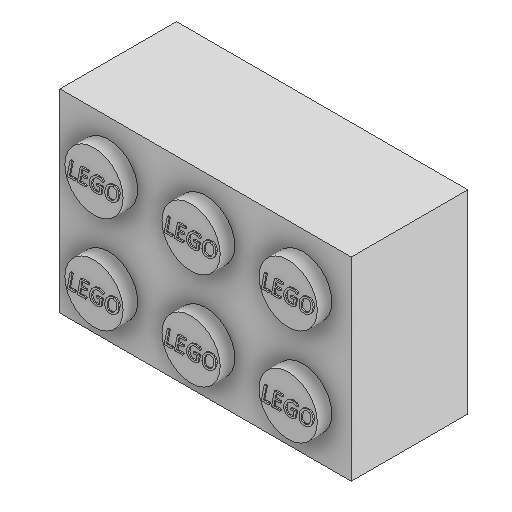
# Autodesk Inventor part: LEGO 2x4 Brick
Saved by Autodesk Inventor 2026.2 (Build 302298000, 298)
## iProperties
Created: 2026-01-06
Part Number: LEGO 2x4 Brick
Material: Generic
Document SubType Name: Modeling
Designer: andyeske
Density: 1 g/cm^3
Appearance: Default
Author: andyeske
Autodesk Inventor part; units mm, degrees
ref_plane "YZ Plane" through (0, 0, 0) normal (1, 0, 0) x (0, 1, 0)
ref_plane "XZ Plane" through (0, 0, 0) normal (0, 1, 0) x (-1, 0, 0)
ref_plane "XY Plane" through (0, 0, 0) normal (0, 0, 1) x (1, 0, 0)
sketch "Sketch1" plane through (0, 0, 0) normal (0, 0, 1) x (1, 0, 0)
  line L0 (-12, -8) -> (12, -8)
  line L1 (12, -8) -> (12, 8)
  line L2 (12, 8) -> (-12, 8)
  line L3 (-12, 8) -> (-12, -8)
  line L4 (-12, -8) -> (12, 8) construction
  line L5 (12, -8) -> (-12, 8) construction
  point P0 (0, 0)
  dimension "d0" = 24
  dimension "d1" = 16
  constraints: 12 end point, 2 midpoint, 2 parallel, 1 horizontal, 1 perpendicular
  measures "d0" distance of L1.end L2.end
  measures "d1" distance of L0.end L1.end
extrude "Extrusion1" add sketch "Sketch1" along normal blind 9.6
shell "Shell1" thickness 1.2 removed faces 1 at (4, -2.6667, 0)
sketch "Sketch2" plane through (0, 0, 9.6) normal (0, 0, 1) x (1, 0, 0)
  line L0 (-12, 4) -> (-8, 4) construction
  line L1 (-8, 4) -> (-8, 8) construction
  line L2 (-12, 8) -> (-12, -8) projected
  line L3 (12, 8) -> (-12, 8) projected
  circle A0 centre (-8, 4) radius 2.4
  point P0 (0, 0)
  dimension "d5" = 4
  dimension "d6" = 4
  dimension "d7" = 4.8
  constraints: 4 end point, 2 point on line, 1 centre point, 1 coincident, 1 horizontal, 1 perpendicular
  measures "d5" distance of L0.end L1.end
  measures "d6" distance of L0.start L0.end
  measures "d7" diameter of A0
extrude "Extrusion2" add sketch "Sketch2" along normal blind 1.2
sketch "Sketch3" plane through (-8, 4, 10.8) normal (0, 0, 1) x (1, 0, 0)
  circle A0 centre (0, 0) radius 2.4 projected
  line L0 (-2.3103, -0.65) -> (2.3103, -0.65) construction
  line L1 (0, 0) -> (0, -0.65) construction
  spline S0 degree 2 poles (-1.4435, -0.5379) (-1.4435, -0.5427) (-1.4459, -0.5641) (-1.4519, -0.5892) (-1.4578, -0.6154) (-1.4697, -0.6369) (-1.4852, -0.65) (-1.4948, -0.65) knots 0 0 0 1 2 3 4 5 6 6 6
  line L2 (-1.4948, -0.65) -> (-2.0553, -0.65)
  spline S1 degree 2 poles (-2.0553, -0.65) (-2.0672, -0.65) (-2.0875, -0.6428) (-2.103, -0.6262) (-2.1089, -0.5999) (-2.1041, -0.582) knots 0 0 0 1 2 3 4 4 4
  line L3 (-2.1041, -0.582) -> (-1.8704, 0.5902)
  spline S2 degree 2 poles (-1.8704, 0.5902) (-1.8692, 0.5962) (-1.8573, 0.6081) (-1.8358, 0.6152) (-1.8024, 0.62) (-1.7798, 0.62) knots 0 0 0 1 2 3 4 4 4
  spline S3 degree 2 poles (-1.7798, 0.62) (-1.7559, 0.62) (-1.7237, 0.6152) (-1.7059, 0.6081) (-1.6999, 0.5962) (-1.7023, 0.5902) knots 0 0 0 1 2 3 4 4 4
  line L4 (-1.7023, 0.5902) -> (-1.9205, -0.5045)
  line L5 (-1.9205, -0.5045) -> (-1.4674, -0.5045)
  spline S4 degree 2 poles (-1.4674, -0.5045) (-1.4542, -0.5045) (-1.4435, -0.5224) (-1.4435, -0.5379) knots 0 0 0 1 2 2 2
  spline S5 degree 2 poles (-0.3405, 0.5818) (-0.3405, 0.5771) (-0.3416, 0.5568) (-0.3464, 0.5329) (-0.3536, 0.5079) (-0.3643, 0.4876) (-0.381, 0.4745) (-0.3917, 0.4745) knots 0 0 0 1 2 3 4 5 6 6 6
  line L6 (-0.3917, 0.4745) -> (-0.8842, 0.4745)
  line L7 (-0.8842, 0.4745) -> (-0.9641, 0.0774)
  line L8 (-0.9641, 0.0774) -> (-0.5396, 0.0774)
  spline S6 degree 2 poles (-0.5396, 0.0774) (-0.5277, 0.0774) (-0.5158, 0.0619) (-0.5158, 0.0464) knots 0 0 0 1 2 2 2
  spline S7 degree 2 poles (-0.5158, 0.0464) (-0.5158, 0.0416) (-0.5181, 0.0202) (-0.5229, -0.0037) (-0.5301, -0.0275) (-0.5408, -0.0454) (-0.5563, -0.0585) (-0.567, -0.0585) knots 0 0 0 1 2 3 4 5 6 6 6
  line L9 (-0.567, -0.0585) -> (-0.9916, -0.0585)
  line L10 (-0.9916, -0.0585) -> (-1.0822, -0.5105)
  line L11 (-1.0822, -0.5105) -> (-0.5801, -0.5105)
  spline S8 degree 2 poles (-0.5801, -0.5105) (-0.5706, -0.5105) (-0.5575, -0.526) (-0.5575, -0.5427) knots 0 0 0 1 2 2 2
  spline S9 degree 2 poles (-0.5575, -0.5427) (-0.5575, -0.5486) (-0.5599, -0.5701) (-0.5646, -0.594) (-0.5706, -0.6178) (-0.5825, -0.6381) (-0.5992, -0.65) (-0.6088, -0.65) knots 0 0 0 1 2 3 4 5 6 6 6
  line L12 (-0.6088, -0.65) -> (-1.2169, -0.65)
  spline S10 degree 2 poles (-1.2169, -0.65) (-1.2277, -0.65) (-1.2479, -0.6428) (-1.2622, -0.6262) (-1.2682, -0.5999) (-1.2634, -0.582) knots 0 0 0 1 2 3 4 4 4
  line L13 (-1.2634, -0.582) -> (-1.0381, 0.5461)
  spline S11 degree 2 poles (-1.0381, 0.5461) (-1.0309, 0.5842) (-0.9844, 0.614) (-0.9617, 0.614) knots 0 0 0 1 2 2 2
  line L14 (-0.9617, 0.614) -> (-0.3631, 0.614)
  spline S12 degree 2 poles (-0.3631, 0.614) (-0.3405, 0.614) (-0.3405, 0.5818) knots 0 0 0 1 1 1
  spline S13 degree 2 poles (0.8723, 0.4769) (0.8723, 0.4697) (0.8699, 0.4495) (0.864, 0.4268) (0.8568, 0.403) (0.8473, 0.3839) (0.8353, 0.3732) (0.8282, 0.3732) knots 0 0 0 1 2 3 4 5 6 6 6
  spline S14 degree 2 poles (0.8282, 0.3732) (0.8139, 0.3732) (0.7638, 0.4089) (0.6803, 0.4531) (0.5611, 0.4888) (0.4788, 0.4888) knots 0 0 0 1 2 3 4 4 4
  spline S15 degree 2 poles (0.4788, 0.4888) (0.3917, 0.4888) (0.2403, 0.4375) (0.1127, 0.3457) (0.0137, 0.2217) (-0.0566, 0.0762) (-0.0924, -0.0836) (-0.0924, -0.1658) knots 0 0 0 1 2 3 4 5 6 6 6
  spline S16 degree 2 poles (-0.0924, -0.1658) (-0.0924, -0.2517) (-0.0423, -0.3841) (0.0519, -0.4735) (0.1842, -0.52) (0.2665, -0.52) knots 0 0 0 1 2 3 4 4 4
  spline S17 degree 2 poles (0.2665, -0.52) (0.3273, -0.52) (0.4585, -0.4914) (0.5158, -0.4628) knots 0 0 0 1 2 2 2
  line L15 (0.5158, -0.4628) -> (0.5885, -0.0967)
  line L16 (0.5885, -0.0967) -> (0.2963, -0.0967)
  spline S18 degree 2 poles (0.2963, -0.0967) (0.2856, -0.0967) (0.2725, -0.08) (0.2725, -0.0645) knots 0 0 0 1 2 2 2
  spline S19 degree 2 poles (0.2725, -0.0645) (0.2725, -0.0573) (0.2749, -0.0347) (0.2808, -0.0108) (0.2892, 0.0118) (0.3011, 0.0309) (0.3154, 0.0416) (0.3238, 0.0416) knots 0 0 0 1 2 3 4 5 6 6 6
  line L17 (0.3238, 0.0416) -> (0.7256, 0.0416)
  spline S20 degree 2 poles (0.7256, 0.0416) (0.7531, 0.0416) (0.7769, 0.0047) (0.7709, -0.0263) knots 0 0 0 1 2 2 2
  line L18 (0.7709, -0.0263) -> (0.6732, -0.5141)
  spline S21 degree 2 poles (0.6732, -0.5141) (0.6696, -0.5319) (0.6565, -0.5546) (0.6493, -0.5629) knots 0 0 0 1 2 2 2
  spline S22 degree 2 poles (0.6493, -0.5629) (0.6398, -0.5725) (0.5682, -0.6059) (0.4597, -0.6417) (0.3238, -0.6679) (0.2498, -0.6679) knots 0 0 0 1 2 3 4 4 4
  spline S23 degree 2 poles (0.2498, -0.6679) (0.1222, -0.6679) (-0.071, -0.6023) (-0.2021, -0.4771) (-0.2701, -0.2994) (-0.2701, -0.1873) knots 0 0 0 1 2 3 4 4 4
  spline S24 degree 2 poles (-0.2701, -0.1873) (-0.2701, -0.0824) (-0.2224, 0.1203) (-0.1318, 0.3016) (-0.0006, 0.4554) (0.1711, 0.5675) (0.3762, 0.6319) (0.4955, 0.6319) knots 0 0 0 1 2 3 4 5 6 6 6
  spline S25 degree 2 poles (0.4955, 0.6319) (0.5635, 0.6319) (0.6827, 0.6081) (0.7769, 0.5735) (0.8413, 0.5329) (0.864, 0.5115) (0.8723, 0.4912) (0.8723, 0.4769) knots 0 0 0 1 2 3 4 5 6 6 6
  spline S26 degree 2 poles (2.153, 0.1907) (2.153, 0.1156) (2.1256, -0.0705) (2.0612, -0.2624) (1.9551, -0.4437) (1.7989, -0.5832) (1.5842, -0.6691) (1.4447, -0.6691) knots 0 0 0 1 2 3 4 5 6 6 6
  spline S27 degree 2 poles (1.4447, -0.6691) (1.3338, -0.6691) (1.1657, -0.613) (1.0536, -0.5033) (0.9963, -0.3411) (0.9963, -0.2338) knots 0 0 0 1 2 3 4 4 4
  spline S28 degree 2 poles (0.9963, -0.2338) (0.9963, -0.1503) (1.0261, 0.044) (1.0929, 0.236) (1.2014, 0.4137) (1.3588, 0.552) (1.5699, 0.6331) (1.707, 0.6331) knots 0 0 0 1 2 3 4 5 6 6 6
  spline S29 degree 2 poles (1.707, 0.6331) (1.8179, 0.6331) (1.9837, 0.5759) (2.097, 0.4626) (2.153, 0.298) (2.153, 0.1907) knots 0 0 0 1 2 3 4 4 4
  spline S30 degree 2 poles (1.973, 0.1788) (1.973, 0.2479) (1.942, 0.3624) (1.874, 0.4435) (1.7607, 0.49) (1.6808, 0.49) knots 0 0 0 1 2 3 4 4 4
  spline S31 degree 2 poles (1.6808, 0.49) (1.5795, 0.49) (1.4256, 0.4149) (1.3135, 0.2933) (1.2396, 0.1394) (1.1967, -0.0168) (1.1776, -0.1635) (1.1776, -0.2171) knots 0 0 0 1 2 3 4 5 6 6 6
  spline S32 degree 2 poles (1.1776, -0.2171) (1.1776, -0.2863) (1.2074, -0.3996) (1.2778, -0.4795) (1.391, -0.5236) (1.4721, -0.5236) knots 0 0 0 1 2 3 4 4 4
  spline S33 degree 2 poles (1.4721, -0.5236) (1.5723, -0.5236) (1.7237, -0.4497) (1.8358, -0.3304) (1.9098, -0.179) (1.9539, -0.0239) (1.973, 0.1227) (1.973, 0.1788) knots 0 0 0 1 2 3 4 5 6 6 6
  point P0 (8, -4)
  dimension "d10" = 0.65
  constraints: 4 end point, 2 horizontal, 2 point on circle, 1 midpoint
  measures "d10" distance of L1.start L1.end
extrude "Extrusion3" add sketch "Sketch3" along normal blind 0.1 contours S0 L2 S1 L3 S2 S3 L4 L5 S4 | S5 L6 L7 L8 S6 S7 L9 L10 L11 S8 S9 L12 S10 L13 S11 L14 S12 | S13 S14 S15 S16 S17 L15 L16 S18 S19 L17 S20 L18 S21 S22 S23 S24 S25 | S26 S27 S28 S29
sketch "Sketch4" plane through (10.8, -6.8, 8.4) normal (0, 0, -1) x (-1, 0, 0)
  circle A0 centre (18.8, 10.8) radius 2.4 construction
  circle A1 centre (18.8, 10.8) radius 1.2
  point P0 (10.8, 6.8)
  dimension "d13" = 1.2
  constraints: 1 centre point, 1 coincident
  measures "d13" radial gap between concentric circles of A0 A1
extrude "Extrusion4" cut sketch "Sketch4" against normal blind 1.2
pattern_linear "Rectangular Pattern1" count 3 spacing 8 along (1, 0, 0) count 2 spacing 8 along (0, -1, 0) of "Extrusion3", "Extrusion2", "Extrusion4"
sketch "Sketch5" plane through (10.8, -6.8, 8.4) normal (0, 0, -1) x (-1, 0, 0)
  line L0 (21.6, 13.6) -> (21.6, 0) projected
  line L1 (21.6, 6.8) -> (14.8, 6.8) construction
  line L2 (14.8, 6.8) -> (14.8, 0) construction
  line L3 (21.6, 0) -> (0, 0) projected
  circle A0 centre (14.8, 6.8) radius 3.2
  circle A1 centre (14.8, 6.8) radius 2.6
  point P0 (10.8, 6.8)
  dimension "d22" = 6.8
  dimension "d23" = 6.4
  dimension "d24" = 0.6
  constraints: 4 end point, 3 perpendicular, 2 centre point, 1 coincident, 1 midpoint, 1 point on line
  measures "d22" distance of L1.start L1.end
  measures "d23" diameter of A0
  measures "d24" radial gap between concentric circles of A0 A1
extrude "Extrusion5" add sketch "Sketch5" along normal up to surface (8.4 mm away)
pattern_linear "Rectangular Pattern2" count 2 spacing 8 along (1, 0, 0) of "Extrusion5"
body "Solid1"
